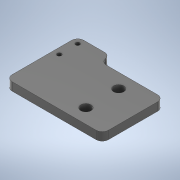
# Autodesk Inventor part: ystop
Saved by Autodesk Inventor 2020.2 (Build 242310000, 310)
## iProperties
Created: 2020-08-09
Part Number: ystop
Material: Generic
Document SubType Name: Modeling
Designer: JK
Density: 1 g/cm^3
Appearance: Smooth - Black
Author: JK
Autodesk Inventor part; units mm, degrees
ref_plane "YZ Plane" through (0, 0, 0) normal (1, 0, 0) x (0, 1, 0)
ref_plane "XZ Plane" through (0, 0, 0) normal (0, 1, 0) x (-1, 0, 0)
ref_plane "XY Plane" through (0, 0, 0) normal (0, 0, 1) x (1, 0, 0)
sketch "Sketch1" plane through (0, 0, 0) normal (0, 1, 0) x (-1, 0, 0)
  line L0 (13, 2.7611) -> (-25, 2.7611)
  line L1 (-25, 2.7611) -> (-25, -27.2389)
  line L2 (-25, -27.2389) -> (13, -27.2389)
  line L3 (13, -27.2389) -> (13, 2.7611)
  circle A0 centre (-10, -4.2389) radius 2.75
  line L4 (-4.8021, -1.4889) -> (-20.6552, -1.4889)
  line L5 (-20.6552, -1.4889) -> (-20.6552, -6.9889)
  line L6 (-20.6552, -6.9889) -> (-4.8021, -6.9889)
  line L7 (-4.8021, -6.9889) -> (-4.8021, -1.4889)
  circle A1 centre (-4.8021, -4.2389) radius 2.75
  circle A2 centre (-20.6552, -4.2389) radius 2.75
  point P0 (0, 0)
  point P1 (-20.6552, -1.4889)
  point P2 (-4.8021, -1.4889)
  point P3 (-10, -6.9889)
  point P4 (-10, -1.4889)
  dimension "d0" = 15
  dimension "d1" = 38
  dimension "d2" = 5.5
  dimension "d3" = 7
  dimension "d4" = 30
  constraints: 16 end point, 4 parallel, 2 horizontal, 2 midpoint, 2 perpendicular, 1 centre point, 1 tangent, 6 other
  measures "d0" distance from line of L1 A0.centre
  measures "d1" distance of L0.start L0.end
  measures "d2" diameter of A0
  measures "d3" distance from line of L0 A0.centre
  measures "d4" distance between parallel lines of L2 L0
extrude "Extrusion1" add sketch "Sketch1" along normal blind 4 contours L3 L2 L1 L0 | A0 A1 L7 | A0 L4 A1 | A1 L6 A0 | A1 L7
sketch "Sketch2" plane through (0, 4, 0) normal (0, 1, 0) x (1, 0, 0)
  line L0 (-13, -2.7611) -> (25, -2.7611) projected
  line L1 (25, -2.7611) -> (34, -2.7611)
  line L2 (34, -2.7611) -> (34, 27.2389)
  line L3 (34, 27.2389) -> (25, 27.2389)
  line L4 (25, 27.2389) -> (25, -2.7611)
  line L5 (25, 27.2389) -> (-13, 27.2389) projected
  point P0 (0, 0)
  dimension "d11" = 9
  constraints: 8 end point, 2 parallel, 1 collinear, 1 horizontal, 1 perpendicular
  measures "d11" distance between parallel lines of L4 L2
extrude "Extrusion2" add sketch "Sketch2" against normal up to surface (4 mm away)
sketch "Sketch3" plane through (0, 4, 0) normal (0, 1, 0) x (1, 0, 0)
  circle A0 centre (20.6552, 20.2389) radius 2.75
  line L0 (34, 27.2389) -> (-13, 27.2389) projected
  arc A1 (20.6552, 1.4889) -> (20.6552, 6.9889) centre (20.6552, 4.2389) ccw projected
  circle A2 centre (10, 20.2389) radius 2.75
  line L1 (10, 17.4889) -> (20.6552, 17.4889)
  line L2 (20.6552, 17.4889) -> (20.6552, 22.9889)
  line L3 (20.6552, 22.9889) -> (10, 22.9889)
  line L4 (10, 22.9889) -> (10, 17.4889)
  point P0 (0, 0)
  point P1 (10, 22.9889)
  point P2 (20.6552, 17.4889)
  dimension "d15" = 5.5
  dimension "d14" = 7
  constraints: 8 end point, 2 parallel, 1 horizontal, 1 perpendicular, 1 vertical alignment, 6 other
  measures "d14" distance from line of L0 point (20.655, 20.239)
extrude "Extrusion3" cut sketch "Sketch3" against normal blind 10
sketch "Sketch4" plane through (0, 4, 0) normal (0, 1, 0) x (1, 0, 0)
  line L0 (-13, 27.2389) -> (-13, -2.7611) projected
  line L1 (-13, 15.4131) -> (3, 15.4131)
  line L2 (3, 15.4131) -> (3, 32.2389)
  line L3 (3, 32.2389) -> (-13, 32.2389)
  line L4 (-13, 32.2389) -> (-13, 15.4131)
  line L5 (34, 27.2389) -> (-13, 27.2389) projected
  point P0 (0, 0)
  point P1 (-13, 27.2389)
  point P2 (3, 27.2389)
  dimension "d18" = 16
  dimension "d19" = 5
  constraints: 8 end point, 2 parallel, 1 horizontal, 1 perpendicular, 1 point on line
  measures "d18" distance between parallel lines of L2 L4
  measures "d19" distance between parallel lines of L5 L3
extrude "Extrusion4" add sketch "Sketch4" against normal up to surface (4 mm away) contours L4 L3 L2 L5
sketch "Sketch5" plane through (0, 4, 0) normal (0, 1, 0) x (1, 0, 0)
  circle A0 centre (-10, 29.2389) radius 1
  circle A1 centre (-10, 20.2389) radius 1
  line L0 (-13, 32.2389) -> (-13, -2.7611) projected
  line L1 (3, 32.2389) -> (-13, 32.2389) projected
  point P0 (0, 0)
  dimension "d22" = 2
  dimension "d23" = 9
  dimension "d24" = 3
  dimension "d25" = 3
  constraints: 2 centre point, 1 equal radius, 1 vertical alignment
  measures "d22" diameter of A0
  measures "d23" distance of A1.centre A0.centre
  measures "d24" distance from line of L0 A0.centre
  measures "d25" distance from line of L1 A0.centre
extrude "Extrusion5" cut sketch "Sketch5" against normal through all
fillet "Fillet1" radius 3 6 edges at (3, 2, -27.2389) (3, 2, -32.2389) (-13, 2, -32.2389) (34, 2, -27.2389) (34, 2, 2.7611) (-13, 2, 2.7611)
sketch "Sketch7" plane through (0, 4, 0) normal (0, 1, 0) x (1, 0, 0)
  arc A0 (10, 6.9889) -> (10, 1.4889) centre (10, 4.2389) ccw projected
  line L0 (10, 6.9889) -> (20.6552, 6.9889) projected
  line L1 (20.6552, 1.4889) -> (10, 1.4889) projected
  arc A1 (20.6552, 1.4889) -> (20.6552, 6.9889) centre (20.6552, 4.2389) ccw projected
  line L2 (20.6552, 17.4889) -> (10, 17.4889) projected
  line L3 (10, 22.9889) -> (20.6552, 22.9889) projected
  arc A2 (10, 22.9889) -> (10, 17.4889) centre (10, 20.2389) ccw projected
  arc A3 (20.6552, 17.4889) -> (20.6552, 22.9889) centre (20.6552, 20.2389) ccw projected
  circle A4 centre (19, 4.2389) radius 2.5
  circle A5 centre (19, 20.2389) radius 2.5
  line L4 (34, 0.2389) -> (34, 24.2389) projected
  point P0 (0, 0)
  dimension "d31" = 5
  dimension "d32" = 15
  constraints: 2 centre point, 2 horizontal alignment, 1 equal radius, 1 vertical alignment
  measures "d31" diameter of A4
  measures "d32" distance from line of A4.centre L4
extrude "Extrusion7" add sketch "Sketch7" against normal up to surface (4 mm away)
body "Solid1"
